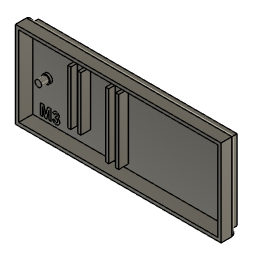
M3 Reference Caliper From 25 v2 (Autodesk Fusion 360 design; units mm, degrees)
Autodesk Fusion 360 part; units mm, degrees
note: some values were not read from the file. Chosen so that the rebuilt part matches the saved one: which bodies a step acts on; which pieces of a blend or face edit are solid. Set by a fixed rule: which sketch regions a step uses; which face or edge a step refers to.
sketch "Schizzo1" plane through (0, 0, 0) normal (0, 1, 0) x (1, 0, 0)
  line L0 (-43.0702, -47.1256) -> (51.9298, -47.1256)
  line L1 (51.9298, -47.1256) -> (51.9298, -7.1256)
  line L2 (51.9298, -7.1256) -> (-43.0702, -7.1256)
  line L3 (-43.0702, -7.1256) -> (-43.0702, -47.1256)
  line L4 (-30.3023, -38.8041) -> (-26.3131, -38.8041) construction
  line L5 (-26.3131, -38.8041) -> (-26.3131, -44.4214) construction
  line L6 (-26.3131, -44.4214) -> (-30.3023, -44.4214) construction
  line L7 (-30.3023, -44.4214) -> (-30.3023, -38.8041) construction
  line L8 (-11.444, -38.8041) -> (-6.602, -38.8041) construction
  line L9 (-6.602, -38.8041) -> (-6.602, -44.4214) construction
  line L10 (-6.602, -44.4214) -> (-11.444, -44.4214) construction
  line L11 (-11.444, -44.4214) -> (-11.444, -38.8041) construction
  line L12 (-14.8624, -15.8255) -> (-20.8624, -15.8255)
  line L13 (-19.4624, -15.8255) -> (-16.2624, -40.8255) construction
  line L14 (-16.2624, -15.8255) -> (-19.4624, -15.8255)
  line L15 (-16.2624, -40.8255) -> (-16.2624, -15.8255)
  line L16 (-19.4624, -15.8255) -> (-19.4624, -40.8255)
  line L17 (-16.2624, -15.8255) -> (-19.4624, -40.8255) construction
  line L18 (-17.8624, -40.8255) -> (-17.8624, -15.8255) construction
  line L19 (-20.8624, -40.8255) -> (-14.8624, -40.8255)
  line L20 (-20.8624, -15.8255) -> (-20.8624, -40.8255)
  line L21 (-14.8624, -40.8255) -> (-14.8624, -15.8255)
  line L22 (-19.4624, -40.8255) -> (-16.2624, -40.8255)
  line L23 (1.2, -40.8255) -> (1.2, -10.8255)
  line L24 (-3.4, -10.8255) -> (-3.4, -40.8255)
  line L25 (2.6, -40.8255) -> (2.6, -10.8255)
  line L26 (-3.4, -40.8255) -> (2.6, -40.8255)
  line L27 (1.2, -10.8255) -> (-2, -40.8255) construction
  line L28 (1.2, -10.8255) -> (-2, -10.8255)
  line L29 (-2, -10.8255) -> (-2, -40.8255)
  line L30 (-2, -10.8255) -> (1.2, -40.8255) construction
  line L31 (2.6, -10.8255) -> (-3.4, -10.8255)
  line L32 (-0.4, -40.8255) -> (-0.4, -10.8255) construction
  line L33 (-2, -40.8255) -> (1.2, -40.8255)
  line L34 (-43.0702, -40.8255) -> (51.9298, -40.8255) construction
  line L35 (-43.0702, -44.4214) -> (51.9298, -44.4214) construction
  line L36 (50.4298, -45.6256) -> (50.4298, -8.6256)
  line L37 (50.4298, -8.6256) -> (-41.5702, -8.6256)
  line L38 (-41.5702, -8.6256) -> (-41.5702, -45.6256)
  line L39 (-41.5702, -45.6256) -> (50.4298, -45.6256)
  line L40 (-38, -10) -> (-25, -10) construction
  line L41 (-25, -10) -> (-25, -15) construction
  line L42 (-25, -15) -> (-38, -15) construction
  line L43 (-38, -15) -> (-38, -10) construction
  line L44 (-43.0702, -38.8041) -> (50.4298, -38.8041) construction
  circle A0 centre (-34.5027, -26.6889) radius 1.5
  circle A1 centre (-34.5027, -26.6889) radius 2
  point P0 (-17.8624, -28.3255)
  point P1 (-0.4, -25.8255)
  point P2 (17.6001, -26.9425)
  dimension "d1" = 40
  dimension "d3" = 5
  dimension "d4" = 5
  dimension "d21" = 6
  dimension "d22" = 25
  dimension "d23" = 3.2
  dimension "d24" = 6
  dimension "d25" = 30
  dimension "d26" = 3.2
  dimension "d33" = 95
  dimension "d34" = -1.5
  dimension "d37" = 5
  dimension "d40" = 3
  dimension "d41" = 4
  text T0 "25" font "Arial" height 5 bold align left top in box 3.9891 x 5.6173 at (-30.3023, -38.8041) x (1, 0) y (0, -1) spacing 1
  text T1 "30" font "Arial" height 5 bold align left top in box 4.842 x 5.6173 at (-11.444, -38.8041) x (1, 0) y (0, -1) spacing 1
  text T2 "M3" font "Arial" height 5 bold align left top in box 13 x 5 at (-38, -10) x (1, 0) y (0, -1) spacing 1
  constraint horizontal L0
  constraint vertical L1
  constraint horizontal L2
  constraint vertical L3
  constraint horizontal L19
  constraint vertical L21
  constraint horizontal L12
  constraint vertical L20
  constraint midpoint L18.start L19
  constraint midpoint L18.end L12
  constraint horizontal L14
  constraint perpendicular L14 L16
  constraint parallel L14 L22
  constraint parallel L15 L16
  constraint coincident P0 L17
  constraint coincident P0 L13
  constraint coincident L14.start L12
  constraint midpoint P0 L18
  constraint horizontal L26
  constraint vertical L25
  constraint horizontal L31
  constraint vertical L24
  constraint midpoint L32.start L26
  constraint midpoint L32.end L31
  constraint horizontal L28
  constraint perpendicular L28 L29
  constraint parallel L28 L33
  constraint parallel L23 L29
  constraint coincident P1 L27
  constraint coincident P1 L30
  constraint coincident L23.end L31
  constraint midpoint P1 L32
  constraint coincident L3 L34.start
  constraint coincident L1 L34.end
  constraint perpendicular L1 L34
  constraint collinear L26 L34
  constraint coincident L3 L35.start
  constraint coincident L1 L35.end
  constraint perpendicular L1 L35
  constraint collinear L19 L34
  constraint collinear L6 L35
  constraint collinear L10 L35
  constraint coincident L3 L44.start
  constraint coincident L36 L44.end
  constraint perpendicular L36 L44
  constraint collinear L4 L44
  constraint collinear L8 L44
  constraint concentric A0 A1
  measures "d1" distance of L0 L2
  measures "d21" distance of L19.start L19.end
  measures "d22" distance of L19.start L12.end
  measures "d23" distance of L15 L16
  measures "d24" distance of L24.end L25.start
  measures "d25" distance of L24.start L24.end
  measures "d26" distance of L23 L29
  measures "d33" distance of L1 L3
  measures "d40" diameter of A0
  measures "d41" diameter of A1
extrude "Estrusione1" add sketch "Schizzo1" along normal blind 0.4 text T0 T1 T2 makes body 1 at (-9.4616, 0, 42.1146) makes body 2 at (-28.697, 0, 39.7181) makes body 3 at (-25.6456, 0, 42.9037) makes body 4 at (-30.4309, 0, 12.6932) makes body 5 at (-37.6874, 0, 12.9786) makes body 6 at (-4.6262, 0, 41.5323)
extrude "Estrusione2" add sketch "Schizzo1" along normal blind 0.5 separate body contours L0 L1 L2 L3 | L12 L15 L19 L21 | L12 L14 L15 L16 L19 L22 | L12 L16 L19 L20 | L23 L26 L28 L29 L31 L33 | L23 L25 L26 L31 | L24 L26 L29 L31 | L36 L37 L38 L39 | A0 | A1 makes body 7
extrude "Estrusione7" cut sketch "Schizzo1" along normal blind 0.4 text T0 T1 T2 bodies 7
extrude "Estrusione6" add sketch "Schizzo1" against normal blind 6.5 contours L0 L1 L2 L3 bodies 7
extrude "Estrusione4" add sketch "Schizzo1" against normal blind 4.5 contours L12 L15 L19 L21 | L12 L14 L15 L16 L19 L22 | L12 L16 L19 L20 | L23 L26 L28 L29 L31 L33 | L23 L25 L26 L31 | L24 L26 L29 L31 | A0 bodies 7
extrude "Estrusione8" add sketch "Schizzo1" against normal blind 1 contours A1 bodies 7
extrude "Estrusione5" cut sketch "Schizzo1" along normal blind 3 from surface at -4.5 contours L12 L14 L15 L16 L19 L22 | L23 L26 L28 L29 L31 L33 bodies 7
sketch "Schizzo2" plane through (0, 0.5, 0) normal (0, 1, 0) x (-1, 0, 0)
  line L0 (43.0702, 7.1256) -> (43.0702, 47.1256)
  line L1 (43.0702, 47.1256) -> (-51.9298, 47.1256)
  line L2 (-51.9298, 47.1256) -> (-51.9298, 7.1256)
  line L3 (-51.9298, 7.1256) -> (43.0702, 7.1256)
  line L4 (-51.9298, 47.1256) -> (43.0702, 47.1256) construction
  line L5 (43.0702, 47.1256) -> (43.0702, 7.1256) construction
  line L6 (43.0702, 7.1256) -> (-51.9298, 7.1256) construction
  line L7 (-51.9298, 7.1256) -> (-51.9298, 47.1256) construction
  line L8 (43.0702, 47.1256) -> (-51.9298, 47.1256) construction
  line L9 (-51.9298, 47.1256) -> (-51.9298, 7.1256) construction
  line L10 (-51.9298, 7.1256) -> (43.0702, 7.1256) construction
  line L11 (43.0702, 7.1256) -> (43.0702, 47.1256) construction
  line L12 (-51.9298, 27.1256) -> (-50, 27.1256) construction
  line L13 (-50, 27.1256) -> (43.0702, 27.1256) construction
  line L14 (-4.4298, 47.1256) -> (-4.4298, 7.1256) construction
  line L15 (41.4702, 8.7256) -> (-50.3298, 8.7256)
  line L16 (-50.3298, 8.7256) -> (-50.3298, 45.5256)
  line L17 (-50.3298, 45.5256) -> (41.4702, 45.5256)
  line L18 (41.4702, 45.5256) -> (41.4702, 8.7256)
  line L19 (41.4702, 8.7256) -> (-50.3298, 45.5256) construction
  line L20 (-50.3298, 8.7256) -> (41.4702, 45.5256) construction
  point P0 (-4.4298, 27.1256)
  dimension "d44" = 1.6
  dimension "d45" = 1.6
  constraint horizontal L4
  constraint vertical L5
  constraint horizontal L6
  constraint vertical L7
  constraint collinear L4 L8
  constraint collinear L7 L9
  constraint collinear L6 L10
  constraint collinear L5 L11
  constraint midpoint L9 L12.start
  constraint perpendicular L9 L12
  constraint midpoint L11 L13.end
  constraint perpendicular L11 L13
  constraint midpoint L4 L14.start
  constraint midpoint L6 L14.end
  constraint horizontal L15
  constraint perpendicular L15 L16
  constraint parallel L15 L17
  constraint parallel L16 L18
  constraint coincident L19 P0
  constraint coincident L20 P0
  constraint midpoint L14 P0
  measures "d44" distance of L7 L16
  measures "d45" distance of L4 L17
extrude "Estrusione9" add sketch "Schizzo2" along normal blind 2 contours L15 L16 L17 L18 bodies 7
fillet "Raccordo1" radius 2 4 edges at (4.4298, 0.5, 7.1256) (51.9298, 0.5, 27.1256) (-43.0702, 0.5, 27.1256) (4.4298, 0.5, 47.1256) on bodies 7
equation "d7 = 6 mm"
equation "d9 = 3.2 mm"
equation "d21 = d7"
equation "d23 = d9"
equation "d24 = d7"
equation "d26 = d9"
equation "d45 = d44"
